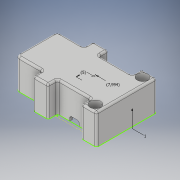
# Autodesk Inventor part: rearcap
Saved by Autodesk Inventor 2019 (Build 230136000, 136)
## iProperties
Created: 2021-01-24
Part Number: rearcap
Material: Genérico
Document SubType Name: Modeling
Designer: Juan M. Casillas
Density: 1 g/cm^3
Appearance: Valor por defecto
Author: Juan M. Casillas
## iProperties of the stored document rearcap_3DPrint.ipt
Created: 2021-01-24
Part Number: rearcap_3DPrint
Material: Genérico
Document SubType Name: Modeling
Designer: Juan M. Casillas
Density: 1 g/cm^3
Appearance: Valor por defecto
Author: Juan M. Casillas
Autodesk Inventor part; units mm, degrees
ref_plane "YZ Plane" through (0, 0, 0) normal (1, 0, 0) x (0, 1, 0)
ref_plane "XZ Plane" through (0, 0, 0) normal (0, 1, 0) x (-1, 0, 0)
ref_plane "XY Plane" through (0, 0, 0) normal (0, 0, 1) x (1, 0, 0)
sketch "Sketch2" plane through (0, 0, 0) normal (0, 1, 0) x (-1, 0, 0)
  circle A0 centre (-1.8699, -7.65) radius 2.825 construction
  circle A1 centre (-1.8699, 17.35) radius 2.825 construction
  arc A2 (-5.8668, -10.15) -> (-4.8668, -11.15) centre (-4.8668, -10.15) ccw
  line L0 (-4.8668, -11.15) -> (1.127, -11.15)
  arc A3 (1.127, -11.15) -> (2.127, -10.15) centre (1.127, -10.15) ccw
  line L1 (2.127, -7.15) -> (2.127, -10.15)
  arc A4 (3.127, -6.15) -> (2.127, -7.15) centre (3.127, -7.15) ccw
  line L2 (3.127, -6.15) -> (14.3101, -6.15)
  arc A5 (14.3101, -6.15) -> (16.3101, -4.15) centre (14.3101, -4.15) ccw
  line L3 (16.3101, -4.15) -> (16.3101, 13.85)
  arc A6 (16.3101, 13.85) -> (14.3101, 15.85) centre (14.3101, 13.85) ccw
  line L4 (14.3101, 15.85) -> (3.127, 15.85)
  arc A7 (2.127, 16.85) -> (3.127, 15.85) centre (3.127, 16.85) ccw
  line L5 (2.127, 16.85) -> (2.127, 19.85)
  arc A8 (2.127, 19.85) -> (1.127, 20.85) centre (1.127, 19.85) ccw
  line L6 (-4.8668, 20.85) -> (1.127, 20.85)
  arc A9 (-4.8668, 20.85) -> (-5.8668, 19.85) centre (-4.8668, 19.85) ccw
  line L7 (-5.8668, 16.85) -> (-5.8668, 19.85)
  arc A10 (-6.8668, 15.85) -> (-5.8668, 16.85) centre (-6.8668, 16.85) ccw
  arc A11 (-5.8668, -7.15) -> (-6.8668, -6.15) centre (-6.8668, -7.15) ccw
  line L8 (-5.8668, -7.15) -> (-5.8668, -10.15)
  circle A12 centre (14.3101, 13.85) radius 1.475 construction
  circle A13 centre (14.3101, -4.15) radius 1.475 construction
  line L9 (2.05, -0.05) -> (-26.5382, -0.05) construction
  line L10 (-26.5382, -0.05) -> (-26.5382, 9.75) construction
  line L11 (-26.5382, 9.75) -> (2.05, 9.75) construction
  line L12 (2.05, 9.75) -> (2.05, -0.05) construction
  arc A14 (3.127, -6.15) -> (2.127, -7.15) centre (3.127, -7.15) ccw construction
  line L13 (3.127, -6.15) -> (-7.6134, -6.15) construction
  line L14 (2.127, -7.15) -> (2.127, -10.15) construction
  line L15 (2.127, -8.65) -> (-28.0746, -8.65) construction
  line L16 (-27.4996, -5.5642) -> (-27.4996, -10.2603) construction
  line L17 (-24.5026, -11.15) -> (-30.4966, -11.15)
  line L18 (-31.4966, -10.15) -> (-31.4966, -7.15)
  line L19 (-23.5026, -7.15) -> (-23.5026, -10.15)
  line L20 (-23.5026, -11.15) -> (-31.4966, -6.15) construction
  line L21 (-31.4966, -11.15) -> (-23.5026, -6.15) construction
  line L22 (-1.8699, -7.65) -> (-29.7598, -7.65) construction
  line L23 (-27.4996, 15.85) -> (-27.4996, 18.35) construction
  line L24 (-31.4966, 16.85) -> (-31.4966, 19.85)
  line L25 (-30.4966, 20.85) -> (-24.5026, 20.85)
  line L26 (-23.5026, 19.85) -> (-23.5026, 16.85)
  line L27 (-23.5026, 15.85) -> (-31.4966, 20.85) construction
  line L28 (-31.4966, 15.85) -> (-23.5026, 20.85) construction
  line L29 (-1.8699, 17.35) -> (-30.0753, 17.35) construction
  line L30 (-22.5026, -6.15) -> (-6.8668, -6.15)
  line L31 (-22.5026, 15.85) -> (-6.8668, 15.85)
  line L32 (-6.8668, 15.85) -> (-23.5026, 15.85)
  arc A15 (-22.5026, -6.15) -> (-23.5026, -7.15) centre (-22.5026, -7.15) ccw
  arc A16 (-24.5026, -11.15) -> (-23.5026, -10.15) centre (-24.5026, -10.15) ccw
  arc A17 (-31.4966, -10.15) -> (-30.4966, -11.15) centre (-30.4966, -10.15) ccw
  arc A18 (-23.5026, 16.85) -> (-22.5026, 15.85) centre (-22.5026, 16.85) ccw
  arc A19 (-23.5026, 19.85) -> (-24.5026, 20.85) centre (-24.5026, 19.85) ccw
  arc A20 (-30.4966, 20.85) -> (-31.4966, 19.85) centre (-30.4966, 19.85) ccw
  line L33 (-31.4966, -7.15) -> (-31.4966, 16.85)
  point P0 (0, 0)
  point P1 (0, 0)
  point P2 (-27.4996, -8.65)
  point P3 (-27.4996, -7.65)
  point P4 (-27.4996, 17.35)
  point P5 (-27.4996, -7.65)
  dimension "d5" = 5
  dimension "d6" = 7.9938
  dimension "d10" = 1
  constraints: 68 end point, 34 point on circle, 21 centre point, 21 point on line, 14 tangent, 5 equal radius, 5 midpoint, 4 horizontal, 3 perpendicular, 2 parallel, 1 coincident, 1 vertical
  measures "d5" distance between parallel lines of L0 L13
  measures "d6" distance between parallel lines of L8 L1
  measures "d10" radius of A15
extrude "Extrusion1" add sketch "Sketch2" along normal blind 16
sketch "Sketch3" plane through (0, 0, 0) normal (0, -1, 0) x (1, 0, 0)
  arc A0 (5.8668, 16.85) -> (6.8668, 15.85) centre (6.8668, 16.85) ccw projected
  line L0 (5.8668, 16.85) -> (5.8668, 19.85) projected
  arc A1 (5.8668, 19.85) -> (4.8668, 20.85) centre (4.8668, 19.85) ccw projected
  line L1 (4.8668, 20.85) -> (-1.127, 20.85) projected
  arc A2 (-1.127, 20.85) -> (-2.127, 19.85) centre (-1.127, 19.85) ccw projected
  line L2 (-2.127, 19.85) -> (-2.127, 16.85) projected
  arc A3 (-3.127, 15.85) -> (-2.127, 16.85) centre (-3.127, 16.85) ccw projected
  line L3 (-3.127, 15.85) -> (-14.3101, 15.85) projected
  arc A4 (-14.3101, 15.85) -> (-16.3101, 13.85) centre (-14.3101, 13.85) ccw projected
  line L4 (-16.3101, 13.85) -> (-16.3101, -4.15) projected
  arc A5 (-16.3101, -4.15) -> (-14.3101, -6.15) centre (-14.3101, -4.15) ccw projected
  line L5 (-14.3101, -6.15) -> (-3.127, -6.15) projected
  arc A6 (-2.127, -7.15) -> (-3.127, -6.15) centre (-3.127, -7.15) ccw projected
  line L6 (-2.127, -7.15) -> (-2.127, -10.15) projected
  arc A7 (-2.127, -10.15) -> (-1.127, -11.15) centre (-1.127, -10.15) ccw projected
  line L7 (-1.127, -11.15) -> (4.8668, -11.15) projected
  arc A8 (4.8668, -11.15) -> (5.8668, -10.15) centre (4.8668, -10.15) ccw projected
  line L8 (5.8668, -10.15) -> (5.8668, -7.15) projected
  arc A9 (6.8668, -6.15) -> (5.8668, -7.15) centre (6.8668, -7.15) ccw projected
  line L9 (6.8668, -6.15) -> (22.5026, -6.15) projected
  arc A10 (23.5026, -7.15) -> (22.5026, -6.15) centre (22.5026, -7.15) ccw projected
  line L10 (23.5026, -7.15) -> (23.5026, -10.15) projected
  arc A11 (23.5026, -10.15) -> (24.5026, -11.15) centre (24.5026, -10.15) ccw projected
  line L11 (24.5026, -11.15) -> (30.4966, -11.15) projected
  arc A12 (30.4966, -11.15) -> (31.4966, -10.15) centre (30.4966, -10.15) ccw projected
  line L12 (31.4966, -10.15) -> (31.4966, 19.85) projected
  arc A13 (31.4966, 19.85) -> (30.4966, 20.85) centre (30.4966, 19.85) ccw projected
  line L13 (30.4966, 20.85) -> (24.5026, 20.85) projected
  arc A14 (24.5026, 20.85) -> (23.5026, 19.85) centre (24.5026, 19.85) ccw projected
  line L14 (23.5026, 19.85) -> (23.5026, 16.85) projected
  arc A15 (22.5026, 15.85) -> (23.5026, 16.85) centre (22.5026, 16.85) ccw projected
  line L15 (22.5026, 15.85) -> (6.8668, 15.85) projected
  line L16 (-14.3101, 14.45) -> (-3.127, 14.45)
  arc A16 (-3.127, 14.45) -> (-0.727, 16.85) centre (-3.127, 16.85) ccw
  line L17 (-0.727, 16.85) -> (-0.727, 19.45)
  line L18 (-0.727, 19.45) -> (4.4668, 19.45)
  line L19 (4.4668, 19.45) -> (4.4668, 16.85)
  arc A17 (4.4668, 16.85) -> (6.8668, 14.45) centre (6.8668, 16.85) ccw
  line L20 (6.8668, 14.45) -> (30.0966, 14.45)
  line L21 (30.0966, 19.45) -> (30.0966, -9.75)
  line L22 (30.0966, -4.75) -> (6.8668, -4.75)
  arc A18 (6.8668, -4.75) -> (4.4668, -7.15) centre (6.8668, -7.15) ccw
  line L23 (4.4668, -7.15) -> (4.4668, -9.75)
  line L24 (4.4668, -9.75) -> (-0.727, -9.75)
  line L25 (-0.727, -9.75) -> (-0.727, -7.15)
  arc A19 (-0.727, -7.15) -> (-3.127, -4.75) centre (-3.127, -7.15) ccw
  line L26 (-3.127, -4.75) -> (-14.3101, -4.75)
  arc A20 (-14.9101, -4.15) -> (-14.3101, -4.75) centre (-14.3101, -4.15) ccw
  line L27 (-14.9101, -4.15) -> (-14.9101, 13.85)
  arc A21 (-14.3101, 14.45) -> (-14.9101, 13.85) centre (-14.3101, 13.85) ccw
  point P0 (0, 0)
  dimension "d13" = 1.4
  constraints: 24 end point, 12 point on circle, 6 centre point, 2 point on line, 13 other
  measures "d13" distance between parallel lines of L3 L16
extrude "Extrusion2" cut sketch "Sketch3" against normal blind 15.6 contours L16 A16 L17 L18 L19 A17 L20 L21 L22 A18 L23 L24 L25 A19 L26 A20 L27 A21
fillet "Fillet1" radius 1 20 edges at (30.0966, 7.8, 14.45) (30.0966, 7.8, -4.75) (18.4817, 15.6, 14.45) (4.4668, 15.6, 18.15) (5.1698, 15.6, 15.1529) (1.8699, 15.6, 19.45) (-0.727, 15.6, 18.15) (-8.7186, 15.6, 14.45) (-14.7344, 15.6, 14.2743) (-14.9101, 15.6, 4.85) (-14.7344, 15.6, -4.5743) (-8.7186, 15.6, -4.75) (-1.43, 15.6, -5.4529) (-0.727, 15.6, -8.45) (-1.43, 15.6, 15.1529) (1.8699, 15.6, -9.75) (4.4668, 15.6, -8.45) (18.4817, 15.6, -4.75) (5.1698, 15.6, -5.4529) (30.0966, 15.6, 4.85)
sketch "Sketch4" plane through (0, 16, 0) normal (0, 1, 0) x (1, 0, 0)
  point P0 (0, 0)
  point P1 (27.4996, -17.35)
  point P2 (27.4996, 7.65)
hole "Hole1" at (27.4996, 16, -7.65) at (27.4996, 16, 17.35) direction (0, -1, 0) diameter 5.65 depth 13
hole "Hole2" at (27.4996, 0, 17.35) at (27.4996, 0, -7.65) direction (0, 1, 0) diameter 2.95 end through all
sketch "Sketch5" plane through (6.8668, 0, 15.85) normal (0, 0, 1) x (1, 0, 0)
  line L0 (-4.9969, 0) -> (23.2085, 0) construction
  line L1 (15.6358, 0) -> (0, 0) construction
  line L2 (8.011, 0) -> (8.011, 5.1734) construction
  line L3 (5.511, 2.5) -> (10.511, 2.5)
  line L4 (10.511, 2.5) -> (10.511, -2.5)
  line L5 (10.511, -2.5) -> (5.511, -2.5) construction
  line L6 (5.511, -2.5) -> (5.511, 2.5)
  line L7 (5.511, 2.5) -> (10.511, -2.5) construction
  line L8 (10.511, 2.5) -> (5.511, -2.5) construction
  line L9 (5.511, 0) -> (10.511, 0)
  point P0 (-6.8668, 0)
  dimension "d31" = 5
  dimension "d32" = 5
  constraints: 16 end point, 4 midpoint, 2 parallel, 2 perpendicular, 1 horizontal, 1 point on line
  measures "d31" distance of L4.end L5.end
  measures "d32" distance of L3.end L4.end
extrude "Extrusion3" cut sketch "Sketch5" against normal blind 3
fillet "Fillet2" radius 1 2 edges at (12.3778, 2.5, 15.15) (17.3778, 2.5, 15.15)
sketch "Sketch6" plane through (22.5026, 0, -6.15) normal (0, 0, -1) x (-1, 0, 0)
  line L0 (5.1248, 0) -> (5.1248, 1.5) projected
  arc A0 (6.1248, 2.5) -> (5.1248, 1.5) centre (6.1248, 1.5) ccw projected
  line L1 (6.1248, 2.5) -> (9.1248, 2.5) projected
  arc A1 (10.1248, 1.5) -> (9.1248, 2.5) centre (9.1248, 1.5) ccw projected
  line L2 (10.1248, 1.5) -> (10.1248, 0) projected
  line L3 (10.1248, 0) -> (5.1248, 0)
  line L4 (-6.594, 0) -> (15.6358, 0) projected
  point P0 (22.5026, 0)
  constraints: 2 end point, 1 collinear
extrude "Extrusion4" cut sketch "Sketch6" against normal blind 3
fillet "Fillet3" radius 1 32 edges at (-15.7243, 16, 15.2642) (-8.7186, 16, 15.85) (-2.4199, 16, 16.1429) (-2.127, 16, 18.35) (-1.8341, 16, 20.5571) (1.8699, 16, 20.85) (5.5739, 16, 20.5571) (5.8668, 16, 18.35) (6.1597, 16, 16.1429) (14.6847, 16, 15.85) (23.2097, 16, 16.1429) (23.5026, 16, 18.35) (23.7955, 16, 20.5571) (27.4996, 16, 20.85) (31.2037, 16, 20.5571) (31.4966, 16, 4.85) (31.2037, 16, -10.8571) (27.4996, 16, -11.15) (23.7955, 16, -10.8571) (23.5026, 16, -8.65) (23.2097, 16, -6.4429) (14.6847, 16, -6.15) (6.1597, 16, -6.4429) (5.8668, 16, -8.65) (5.5739, 16, -10.8571) (1.8699, 16, -11.15) (-1.8341, 16, -10.8571) (-2.127, 16, -8.65) (-2.4199, 16, -6.4429) (-8.7186, 16, -6.15) (-15.7243, 16, -5.5642) (-16.3101, 16, 4.85)
equation "\"d9\" = d8"
equation "\"d8\" = 2.5"
body "Solid1"
